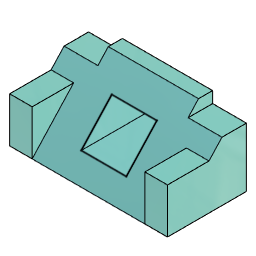
Exercise-17 v1 (Autodesk Fusion 360 design; units mm, degrees)
Autodesk Fusion 360 part; units mm, degrees
sketch "Sketch1" plane through (0, 0, 0) normal (0, 0, 1) x (1, 0, 0)
box "BoxPrimitive1" add length 28 width 56 height 25 placed x (0, 1, 0) y (-1, 0, 0) z (0, 0, 1) at (56, 0, 0)
sketch "Sketch2" plane through (56, 0, 0) normal (1, 0, 0) x (0, 1, 0)
  line L0 (0, 25) -> (0, 0)
  line L1 (0, 0) -> (28, 0)
  line L2 (28, 0) -> (28, 25)
  line L3 (28, 25) -> (0, 25)
  line L4 (0, 0) -> (23, 25)
  line L5 (28, 21) -> (19.32, 21)
  line L6 (0, 16) -> (14.72, 16)
  dimension "d6" = 5
  dimension "d7" = 16
  dimension "d8" = 5
  constraint coincident L0.end L1.start
  constraint coincident L3 L4.end
  constraint coincident L2 L5.start
  constraint coincident L4 L5.end
  constraint perpendicular L2 L5
  constraint coincident L0 L6.start
  constraint coincident L4 L6.end
  constraint perpendicular L0 L6
  measures "d6" distance of L2.end L4.end
  measures "d7" distance of L0.end L6.start
  measures "d8" vertical distance of L5.end L6.end
extrude "Extrude1" cut sketch "Sketch2" against normal blind 56 contours L0 L3 L4 L6
extrude "Extrude2" cut sketch "Sketch2" against normal blind 40 from surface at -8 contours L0 L4 L6
extrude "Extrude3" cut sketch "Sketch2" against normal blind 12 contours L2 L3 L4 L5
ref_plane "WorkPlane1" through (28, 14, 12.5) normal (-1, 0, 0) x (0, 0, 1)
mirror "Mirror1" about plane through (28, 14, 12.5) normal (-1, 0, 0) of "Extrude3"
sketch "Sketch3" plane through (0, 0, 0) normal (0, -0.735931, 0.677057) x (1, 0, 0)
  line L0 (12, 28.5353) -> (0, 28.5353)
  line L1 (0, 28.5353) -> (0, 21.7412)
  line L2 (0, 21.7412) -> (8, 21.7412)
  line L3 (8, 21.7412) -> (8, 0)
  line L4 (8, 0) -> (48, 0)
  line L5 (48, 0) -> (48, 21.7412)
  line L6 (48, 21.7412) -> (56, 21.7412)
  line L7 (56, 21.7412) -> (56, 28.5353)
  line L8 (56, 28.5353) -> (44, 28.5353)
  line L9 (44, 28.5353) -> (44, 33.9706)
  line L10 (44, 33.9706) -> (12, 33.9706)
  line L11 (12, 33.9706) -> (12, 28.5353)
  line L12 (20, 24) -> (36, 24)
  line L13 (36, 24) -> (36, 8)
  line L14 (36, 8) -> (20, 8)
  line L15 (20, 8) -> (20, 24)
  dimension "d18" = 16
  dimension "d19" = 16
  dimension "d20" = 8
  dimension "d21" = 12
  constraint horizontal L12
  constraint vertical L13
  constraint horizontal L14
  constraint vertical L15
  measures "d18" distance of L12.start L12.end
  measures "d19" distance of L12.start L14.end
  measures "d20" distance of L4 L14
  measures "d21" distance of L3 L14.end
sketch "Sketch4" plane through (0, 28, 0) normal (0, 1, 0) x (-1, 0, 0)
  line L0 (0, 21) -> (-12, 21)
  line L1 (-12, 21) -> (-12, 25)
  line L2 (-12, 25) -> (-44, 25)
  line L3 (-44, 25) -> (-44, 21)
  line L4 (-44, 21) -> (-56, 21)
  line L5 (-56, 21) -> (-56, 0)
  line L6 (-56, 0) -> (0, 0)
  line L7 (0, 0) -> (0, 21)
  line L8 (-36, 5.8874) -> (-20, 5.8874)
  line L9 (-20, 5.8874) -> (-20, 17.6623)
  line L10 (-36, 17.6623) -> (-36, 5.8874)
  line L11 (-20, 17.6623) -> (-36, 17.6623)
extrude "Extrude4" cut sketch "Sketch4" against normal blind 28 contours L8 L9 L10 L11
